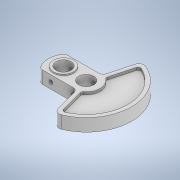
# Autodesk Inventor part: crankshaft counter weight
Saved by Autodesk Inventor 2020 (Build 240168000, 168)
## iProperties
Created: 2020-08-08
Part Number: crankshaft counter weight
Material: Generic
Document SubType Name: Modeling
Designer: benny
Density: 1 g/cm^3
Appearance: Default
Author: benny
Autodesk Inventor part; units mm, degrees
ref_plane "YZ Plane" through (0, 0, 0) normal (1, 0, 0) x (0, 1, 0)
ref_plane "XZ Plane" through (0, 0, 0) normal (0, 1, 0) x (-1, 0, 0)
ref_plane "XY Plane" through (0, 0, 0) normal (0, 0, 1) x (1, 0, 0)
sketch "Sketch2" plane through (0, 0, 0) normal (0, 1, 0) x (-1, 0, 0)
  arc A0 (-9.3175, 34.7733) -> (-9.3175, -34.7733) centre (0, 0) ccw
  line L0 (26.49, 10) -> (-2.6795, 10)
  line L1 (-30, 0) -> (-30, -10)
  line L2 (-2.6795, -10) -> (26.49, -10)
  line L3 (30, -10) -> (30, 0)
  line L4 (30, 10) -> (-30, -10) construction
  line L5 (-30, 10) -> (30, -10) construction
  line L6 (0, 0) -> (-9.3175, 34.7733)
  line L7 (0, 0) -> (48.0971, 0) construction
  line L8 (-12.4484, 0) -> (0, 0)
  line L9 (0, 0) -> (-13.0994, -48.8875)
  line L10 (0, 0) -> (50.6121, 0) construction
  arc A1 (-1.9863, 0.6621) -> (-1.9863, -0.6621) centre (14, 0) ccw
  arc A2 (26.49, -10) -> (26.49, 10) centre (14, 0) ccw
  dimension "d5" = 72
  dimension "d6" = 60
  dimension "d7" = 20
  dimension "d8" = 105
  dimension "d9" = 105
  constraints: 22 end point, 7 point on circle, 7 point on line, 3 centre point, 3 horizontal, 2 midpoint, 2 parallel, 1 coincident, 1 equal length, 1 perpendicular
  measures "d5" diameter of A0
  measures "d6" distance of L3.start L1.end
  measures "d7" distance of L1.end L5.start
  measures "d8" angle of L7 L6
  measures "d9" angle of L9 L10
extrude "Extrusion1" add sketch "Sketch2" along normal blind 10
fillet "Fillet1" radius 4 6 edges at (-26.49, 5, -10) (9.3175, 5, -34.7733) (2.6795, 5, -10) (2.6795, 5, 10) (-26.49, 5, 10) (9.3175, 5, 34.7733)
sketch "Sketch3" plane through (0, 10, 0) normal (0, 1, 0) x (1, 0, 0)
  line L0 (0, 0) -> (-18, 0)
  circle A0 centre (-18, 0) radius 8
  dimension "d14" = 18
  dimension "d15" = 16
  constraints: 2 end point, 1 centre point, 1 coincident, 1 horizontal
  measures "d14" distance of L0.start L0.end
  measures "d15" diameter of A0
extrude "Extrusion2" add sketch "Sketch3" along normal blind 1
sketch "Sketch4" plane through (-18, 11, 0) normal (0, 1, 0) x (1, 0, 0)
  circle A0 centre (0, 0) radius 6
  point P0 (18, 0)
  dimension "d18" = 12
  constraints: 1 centre point
  measures "d18" diameter of A0
extrude "Extrusion3" cut sketch "Sketch4" against normal blind 11
sketch "Sketch5" plane through (0, 0, 0) normal (0, -1, 0) x (1, 0, 0)
  circle A0 centre (0, 0) radius 8
  dimension "d21" = 16
  constraints: 1 centre point, 1 coincident
  measures "d21" diameter of A0
extrude "Extrusion4" add sketch "Sketch5" along normal blind 1
sketch "Sketch6" plane through (0, -1, 0) normal (0, -1, 0) x (1, 0, 0)
  circle A0 centre (0, 0) radius 6
  dimension "d24" = 12
  constraints: 1 centre point, 1 coincident
  measures "d24" diameter of A0
extrude "Extrusion5" cut sketch "Sketch6" against normal blind 11
sketch "Sketch7" plane through (0, 0, 0) normal (0, 0, 1) x (1, 0, 0)
  circle A0 centre (0, 5) radius 1.5
  point P0 (0, 0)
  dimension "d27" = 3
  constraints: 1 centre point
  measures "d27" diameter of A0
extrude "Extrusion6" cut sketch "Sketch7" along normal mid plane 21
sketch "Sketch8" plane through (0, 0, 0) normal (0, 0, 1) x (1, 0, 0)
  circle A0 centre (-18, 5) radius 1.5
  point P0 (0, 0)
  dimension "d30" = 3
  constraints: 1 centre point
  measures "d30" diameter of A0
extrude "Extrusion7" cut sketch "Sketch8" against normal mid plane 21
sketch "Sketch9" plane through (0, 10, 0) normal (0, 1, 0) x (1, 0, 0)
  arc A0 (11.4034, -30.9671) -> (11.4034, 30.9671) centre (0, 0) ccw
  line L0 (3.4739, -12.9647) -> (8.2172, -30.6672) projected
  line L1 (8.2172, 30.6672) -> (3.4739, 12.9647) projected
  arc A1 (5.6369, -9.4459) -> (5.6369, 9.4459) centre (0, 0) ccw
  line L2 (5.6369, 9.4459) -> (11.4034, 30.9671)
  line L3 (11.4034, -30.9671) -> (5.6369, -9.4459)
  line L4 (3.1058, 0) -> (1.7117, 5.2028)
  dimension "d33" = 66
  dimension "d38" = 22
  constraints: 6 end point, 4 point on circle, 3 parallel, 2 centre point, 2 coincident
  measures "d33" diameter of A0
  measures "d38" diameter of A1
extrude "Extrusion8" cut sketch "Sketch9" against normal blind 2
fillet "Fillet3" radius 2 4 edges at (11.4034, 9, 30.9671) (5.6369, 9, 9.4459) (5.6369, 9, -9.4459) (11.4034, 9, -30.9671)
body "Solid1"
